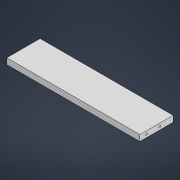
# Autodesk Inventor part: Shelf
Saved by Autodesk Inventor 2021.2 (Build 252289000, 289)
## iProperties
Created: 2021-02-02
Part Number: Shelf
Material: Generic
Document SubType Name: Modeling
Designer: Nedeljko Š
Density: 1 g/cm^3
Appearance: Default
Author: Nedeljko Š
Autodesk Inventor part; units mm, degrees
ref_plane "YZ Plane" through (0, 0, 0) normal (1, 0, 0) x (0, 1, 0)
ref_plane "XZ Plane" through (0, 0, 0) normal (0, 1, 0) x (-1, 0, 0)
ref_plane "XY Plane" through (0, 0, 0) normal (0, 0, 1) x (1, 0, 0)
sketch "Sketch1" plane through (0, 0, 0) normal (0, 1, 0) x (-1, 0, 0)
  line L0 (200, 0) -> (-200, 0)
  line L1 (-200, 0) -> (-200, 100)
  line L2 (-200, 100) -> (200, 100)
  line L3 (200, 100) -> (200, 0)
  point P0 (0, 0)
  point P1 (0, 0)
  dimension "Length" = 400
  dimension "Depth" = 100
  constraints: 8 end point, 2 parallel, 1 coincident, 1 horizontal, 1 midpoint, 1 perpendicular
  measures "Length" distance of L1.end L2.end
  measures "Depth" distance of L0.end L1.end
extrude "Extrusion1" add sketch "Sketch1" along normal mid plane 18
sketch "Sketch2" plane through (200, -9, 100) normal (1, 0, 0) x (0, 0, -1)
  line L0 (0, 0) -> (0, 18) projected
  line L1 (100, 9) -> (100, 18) projected
  point P0 (20, 9)
  point P1 (60, 9)
  point P2 (0, 9)
  dimension "d4" = 20
  dimension "d5" = 40
  constraints: 2 horizontal alignment, 1 midpoint
  measures "d4" distance from line of point (20, 9) L0
  measures "d5" distance from line of point (60, 9) L1
sketch "Sketch3" plane through (0, -9, 0) normal (0, -1, 0) x (1, 0, 0)
  line L0 (200, 0) -> (200, 100) projected
  line L1 (200, 100) -> (-200, 100) projected
  line L2 (0, 0) -> (200, 0) projected
  line L3 (-200, 100) -> (-200, 0) projected
  point P0 (170, 80)
  point P1 (170, 40)
  point P2 (-170, 60)
  point P3 (-170, 20)
  dimension "HoleDepth" = 30
  dimension "d7" = 20
  dimension "d8" = 40
  dimension "d26" = 20
  dimension "d27" = 40
  dimension "d72" = 30
  constraints: 2 vertical alignment
  measures "HoleDepth" distance from line of L0 point (170, 40)
  measures "d7" distance from line of L1 point (170, 80)
  measures "d8" distance from line of L2 point (170, 40)
  measures "d26" distance from line of L2 point (-170, 20)
  measures "d27" distance from line of point (-170, 60) L1
  measures "d72" distance from line of L3 point (-170, 20)
hole "Hole1" at (200, 0, 80) at (200, 0, 40) direction (-1, 0, 0) diameter 6 depth 30
sketch "Sketch4" plane through (-200, -9, 0) normal (-1, 0, 0) x (0, 0, 1)
  line L0 (100, 18) -> (100, 0) projected
  line L1 (0, 0) -> (0, 18) projected
  point P0 (60, 9)
  point P1 (20, 9)
  point P2 (0, 9)
  dimension "d24" = 40
  dimension "d71" = 20
  constraints: 2 horizontal alignment, 1 midpoint
  measures "d24" distance from line of L0 point (60, 9)
  measures "d71" distance from line of point (20, 9) L1
hole "Hole3" at (-200, 0, 60) at (-200, 0, 20) direction (1, 0, 0) diameter 6 depth 30
hole "Hole5" at (170, -9, 80) at (170, -9, 40) direction (0, 1, 0) diameter 15 depth 14
hole "Hole7" at (-170, -9, 60) at (-170, -9, 20) direction (0, 1, 0) diameter 15 depth 14
equation "\"d7\" = d4"
equation "\"d8\" = d5"
equation "\"d26\" = d7"
equation "\"d27\" = d8"
equation "\"d72\" = HoleDepth"
equation "\"d14\" = HoleDepth"
equation "\"d24\" = d5"
equation "\"d71\" = d26"
equation "\"d33\" = HoleDepth"
body "Solid1"
